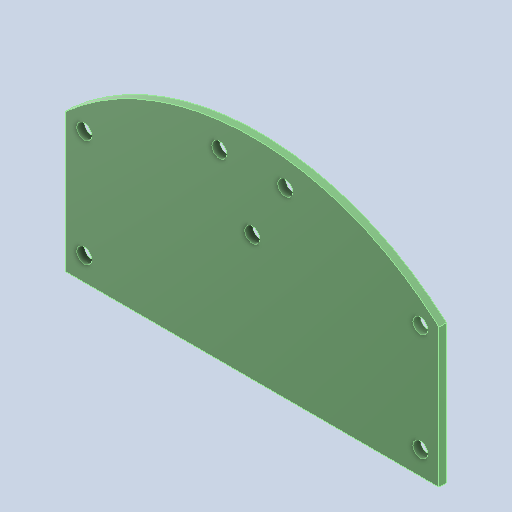
# Autodesk Inventor part: SensorBoard-SPG27
Saved by Autodesk Inventor 2025.3 (Build 293356030, 356C)
## iProperties
Created: 2025-05-29
Part Number: SensorBoard-SPG27
Material: 一般
Document SubType Name: Modeling
Designer: yamashita1
Density: 1 g/cm^3
Appearance: 滑らか - 濃い深緑
Author: yamashita1
Autodesk Inventor part; units mm, degrees
ref_plane "YZ Plane" through (0, 0, 0) normal (1, 0, 0) x (0, 1, 0)
ref_plane "XZ Plane" through (0, 0, 0) normal (0, 1, 0) x (-1, 0, 0)
ref_plane "XY Plane" through (0, 0, 0) normal (0, 0, 1) x (1, 0, 0)
sketch "スケッチ1" plane through (0, 0, 0) normal (0, 0, 1) x (1, 0, 0)
  circle A0 centre (0, 0) radius 60 construction
  line L0 (-40, 60) -> (40, 60) construction
  line L1 (40, 60) -> (40, -60) construction
  line L2 (40, -60) -> (-40, -60) construction
  line L3 (-40, -60) -> (-40, 60) construction
  arc A1 (40, 44.7214) -> (-40, 44.7214) centre (0, 0) ccw
  line L4 (-40, 44.7214) -> (-40, -44.7214)
  line L5 (40, 44.7214) -> (40, -44.7214)
  arc A2 (-40, -44.7214) -> (40, -44.7214) centre (0, 0) ccw
  line L6 (40, -44) -> (-40, -44)
  line L7 (-40, 15) -> (40, 15)
  point P0 (0, 60)
  dimension "d0" = 120
  dimension "d1" = 80
  dimension "d41" = 44
  dimension "d52" = 15
  constraints: 18 end point, 9 point on circle, 8 point on line, 3 centre point, 3 parallel, 3 perpendicular, 2 tangent, 1 coincident, 1 concentric, 1 horizontal, 1 midpoint, 1 vertical, 1 vertical alignment
  measures "d0" diameter of A0
  measures "d1" distance of L1.end L2.end
  measures "d41" distance from line of point (0, 0) L6
  measures "d52" distance from line of L7 point (0, 0)
extrude "基板" add sketch "スケッチ1" along normal blind 1.6 contours L5 L7 L4 A1
sketch "スケッチ3" plane through (0, 0, 1.6) normal (0, 0, 1) x (1, 0, 0)
  line L0 (0, 0) -> (0, 55.332) construction
  line L1 (-15.38, 50) -> (15.38, 50) construction
  line L2 (0, 41.85) -> (-7.0581, 45.925) construction
  line L3 (-7.0581, 45.925) -> (-7.0581, 54.075) construction
  line L4 (-7.0581, 54.075) -> (0, 58.15) construction
  line L5 (0, 58.15) -> (7.0581, 54.075) construction
  line L6 (7.0581, 54.075) -> (7.0581, 45.925) construction
  line L7 (7.0581, 45.925) -> (0, 41.85) construction
  arc A0 (40, 44.7214) -> (-40, 44.7214) centre (0, 0) ccw construction
  point P0 (0, 50)
  point P1 (0, 50)
  point P2 (0, 60)
  dimension "d17" = 16.3
  dimension "d18" = 10
  constraints: 16 end point, 7 coincident, 2 point on line, 1 horizontal, 1 midpoint, 1 point on circle, 1 vertical, 13 other
  measures "d17" distance of L2.start L4.end
  measures "d18" distance from line of point (0, 60) L1
hole "ボールキャスター取付穴" at (-7.0581, 54.075, 1.6) at (7.0581, 54.075, 1.6) at (0, 41.85, 1.6) direction (0, 0, -1) diameter 3.2 end through all
sketch "スケッチ5" plane through (0, 0, 1.6) normal (0, 0, 1) x (1, 0, 0)
  line L0 (0, 0) -> (0, 96.0936) construction
  line L1 (-67.6385, -10) -> (77.8935, -10) construction
  point P0 (-36, 43)
  point P1 (36, 43)
  point P2 (-36, 20)
  point P3 (36, 20)
  dimension "d42" = 72
  dimension "d43" = 10
  dimension "d53" = 23
  dimension "d55" = 43
  constraints: 4 end point, 2 horizontal alignment, 2 vertical alignment, 1 horizontal, 1 symmetric about line, 1 vertical
  measures "d42" distance of point (36, 43) point (-36, 43)
  measures "d43" distance from line of L1 L0.start
  measures "d53" distance of point (-36, 20) point (-36, 43)
  measures "d55" vertical distance of L0.start point (36, 43)
hole "連結穴" at (-36, 43, 1.6) at (36, 43, 1.6) at (-36, 20, 1.6) at (36, 20, 1.6) direction (0, 0, -1) diameter 3.2 end through all
derived "BaseBoard-SPG27.ipt"
equation "\"d42\" = CONN_W"
equation "\"d53\" = CONN_SPAN"
equation "\"d55\" = CONN_L1"
equation "\"CONN_W\" = 72"
equation "\"CONN_SPAN\" = 23"
equation "\"CONN_L1\" = 43"
